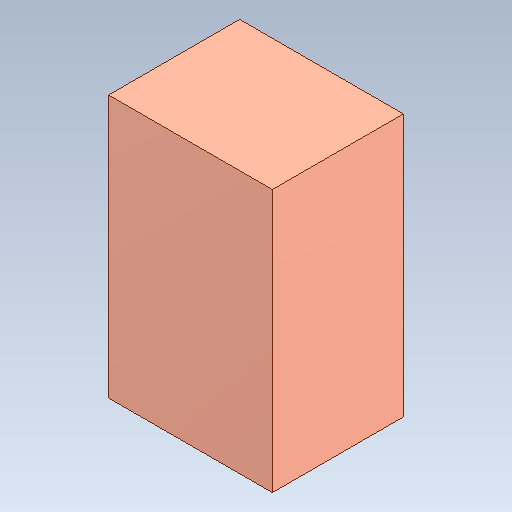
# Autodesk Inventor part: LED1_CHIPLED_0805
Saved by Autodesk Inventor 2021 (Build 250183000, 183)
## iProperties
Created: 2020-11-18
Part Number: LED1_CHIPLED_0805
Material: Generic
Document SubType Name: Modeling
Designer: Admin
Density: 1 g/cm^3
Appearance: CHIPLED_0805, LED1_CHIPLED_0805
Author: Admin
Autodesk Inventor part; units mm, degrees
ref_plane "YZ Plane" through (0, 0, 0) normal (1, 0, 0) x (0, 1, 0)
ref_plane "XZ Plane" through (0, 0, 0) normal (0, 1, 0) x (-1, 0, 0)
ref_plane "XY Plane" through (0, 0, 0) normal (0, 0, 1) x (1, 0, 0)
sketch "CHIPLED_0805, LED1_CHIPLED_0805_29" plane through (0, 0, 0) normal (0, 0, 1) x (1, 0, 0)
  line L0 (-0.625, 1.0038) -> (0.625, 1.0038)
  line L1 (0.625, 1.0038) -> (0.625, -1)
  line L2 (0.625, -1) -> (-0.625, -1)
  line L3 (-0.625, -1) -> (-0.625, 1.0038)
  constraints: 8 end point
extrude "Extrusion1" add sketch "CHIPLED_0805, LED1_CHIPLED_0805_29" along normal blind 1
body "Solid1"
